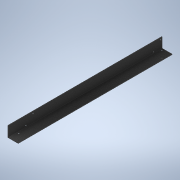
# Autodesk Inventor part: angleline-500
Saved by Autodesk Inventor 2020.4 (Build 244396000, 396)
## iProperties
Created: 2021-02-28
Part Number: angleline-500
Material: Steel
Document SubType Name: Modeling
Designer: AOB
Mass: 518.737 g
Surface Area: 854.662 cm^2
Volume: 66.0811 cm^3
Density: 7.85 g/cm^3
Appearance: Black Cast
Author: AOB
Autodesk Inventor part; units mm, degrees
ref_plane "YZ Plane" through (0, 0, 0) normal (1, 0, 0) x (0, 1, 0)
ref_plane "XZ Plane" through (0, 0, 0) normal (0, 1, 0) x (-1, 0, 0)
ref_plane "XY Plane" through (0, 0, 0) normal (0, 0, 1) x (1, 0, 0)
sketch "Sketch1" plane through (0, 0, 0) normal (0, 0, 1) x (1, 0, 0)
  line L0 (0, 0) -> (0, -38.1)
  line L1 (0, -38.1) -> (38.1, -38.1)
  line L2 (38.1, -38.1) -> (38.1, -36.5125)
  line L3 (38.1, -36.5125) -> (1.5875, -36.5125)
  line L4 (1.5875, -36.5125) -> (1.5875, 0)
  line L5 (1.5875, 0) -> (0, 0)
  dimension "d2" = 1.5875
  dimension "d3" = 1.5875
  dimension "d4" = 38.1
  dimension "d5" = 38.1
  constraints: 12 end point, 5 perpendicular, 1 vertical
  measures "d2" distance of L1.end L2.end
  measures "d3" distance of L4.end L0.start
  measures "d4" distance of L0.start L0.end
  measures "d5" distance of L0.end L1.end
extrude "Extrusion1" add sketch "Sketch1" along normal blind 560
sketch "Sketch2" plane through (0, -38.1, 0) normal (0, -1, 0) x (1, 0, 0)
  line L0 (38.1, 0) -> (1.5875, 0) projected
  line L1 (1.5875, 0) -> (1.5875, 1.5875)
  line L2 (0, 0) -> (0, 560) projected
  line L3 (38.1, 0) -> (38.1, 560) projected
  line L4 (1.5875, 1.5875) -> (38.1, 1.5875)
  line L5 (38.1, 1.5875) -> (38.1, 38.1)
  line L6 (38.1, 38.1) -> (1.5875, 38.1)
  line L7 (1.5875, 38.1) -> (1.5875, 1.5875)
  line L8 (1.5875, 1.5875) -> (38.1, 38.1)
  line L9 (1.5875, 1.5875) -> (6.9757, 6.9757)
  line L10 (1.5875, 521.9) -> (38.1, 521.9)
  line L11 (38.1, 521.9) -> (38.1, 558.4125)
  line L12 (38.1, 558.4125) -> (1.5875, 558.4125)
  line L13 (1.5875, 558.4125) -> (1.5875, 521.9)
  line L14 (1.5875, 521.9) -> (38.1, 558.4125)
  line L15 (1.5875, 521.9) -> (6.9757, 527.2882)
  line L16 (38.1, 560) -> (1.5875, 560) projected
  line L17 (38.1, 560) -> (38.1, 558.4125)
  line L18 (38.1, 558.4125) -> (32.7118, 553.0243)
  line L19 (38.1, 37) -> (28.575, 37)
  line L20 (38.1, 38.1) -> (32.7118, 32.7118)
  point P0 (1.5875, 560)
  dimension "d10" = 36.5125
  dimension "d14" = 1.5875
  dimension "d17" = 7.62
  dimension "d20" = 7.62
  dimension "d21" = 9.525
  dimension "d22" = 7.62
  dimension "d23" = 7.62
  dimension "d38" = 36.5125
  dimension "d39" = 36.5125
  dimension "d40" = 38.1
  dimension "d42" = 1.5875
  dimension "d44" = 1.5875
  constraints: 34 end point, 6 point on line, 5 parallel, 3 horizontal, 2 perpendicular, 1 other
  measures "d10" distance of L6.end L1.end
  measures "d14" distance of L0.end L1.end
  measures "d17" distance of L10.start L15.end
  measures "d20" distance of L11.end L18.end
  measures "d21" distance of L19.start L19.end
  measures "d22" distance of L5.end L20.end
  measures "d23" distance of L1.end L9.end
  measures "d38" distance of L12.end L10.start
  measures "d39" distance of L10.start L10.end
  measures "d40" distance from line of L2 L10.end
  measures "d42" distance from line of L2 L12.end
hole "Hole1" at (32.7118, -38.1, 32.7118) direction (0, 1, 0) diameter 5 end through all
hole "Hole2" at (6.9757, -38.1, 527.2882) at (32.7118, -38.1, 553.0243) at (6.9757, -38.1, 6.9757) direction (0, 1, 0) diameter 5 end through all
sketch "Sketch3" plane through (0, -38.1, 0) normal (-1, 0, 0) x (0, 0, 1)
  line L0 (0, 0) -> (0, 36.5125)
  line L1 (0, 36.5125) -> (1.5875, 36.5125)
  line L2 (0, 38.1) -> (500, 38.1)
  line L3 (0, 0) -> (500, 0)
  line L4 (0, 36.5125) -> (0, 0)
  line L5 (1.5875, 0) -> (38.1, 0)
  line L6 (36.5125, 0) -> (36.5125, 36.5125)
  line L7 (36.5125, 36.5125) -> (0, 36.5125)
  line L8 (0, 36.5125) -> (36.5125, 0)
  line L9 (0, 36.5125) -> (5.3882, 31.1243)
  line L10 (463.4875, 36.5125) -> (463.4875, 0)
  line L11 (463.4875, 0) -> (500, 0)
  line L12 (500, 0) -> (500, 36.5125)
  line L13 (500, 36.5125) -> (463.4875, 36.5125)
  line L14 (463.4875, 36.5125) -> (500, 0)
  line L15 (463.4875, 36.5125) -> (468.8757, 31.1243)
  line L16 (500, 0) -> (500, 36.5125)
  line L17 (500, 0) -> (498.4125, 0)
  line L18 (500, 0) -> (494.6118, 5.3882)
  line L19 (37, 0) -> (37, 9.525) construction
  line L20 (36.5125, 0) -> (31.1243, 5.3882)
  point P0 (0, 38.1)
  dimension "d45" = 36.5125
  dimension "d46" = 1.5875
  dimension "d47" = 7.62
  dimension "d48" = 7.62
  dimension "d49" = 9.525
  dimension "d50" = 7.62
  dimension "d51" = 7.62
  dimension "d52" = 36.5125
  dimension "d53" = 36.5125
  dimension "d54" = 38.1
  dimension "d55" = 1.5875
  dimension "d56" = 0
  constraints: 42 end point, 5 parallel, 5 point on line, 2 perpendicular
  measures "d45" distance of L6.end L4.start
  measures "d46" distance of L1.end L0.end
  measures "d47" distance of L10.start L15.end
  measures "d48" distance of L11.end L18.end
  measures "d49" distance of L19.start L19.end
  measures "d50" distance of L6.start L20.end
  measures "d51" distance of L4.start L9.end
  measures "d52" distance of L12.end L10.start
  measures "d53" distance of L10.start L10.end
  measures "d54" distance from line of L2 L10.end
  measures "d55" distance from line of L2 L12.end
  measures "d56" distance from line of L16 L11.end
hole "Hole3" at (0, -32.7118, 494.6118) at (0, -6.9757, 468.8757) at (0, -6.9757, 5.3882) at (0, -32.7118, 31.1243) direction (1, 0, 0) diameter 5 end through all
equation "\"d10\" = d39"
equation "\"d38\" = d39"
equation "\"d44\" = d42"
equation "\"d45\" = d53"
equation "\"d52\" = d53"
body "Solid1"
